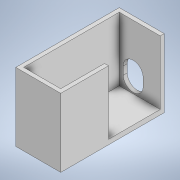
# Autodesk Inventor part: GoProCase
Saved by Autodesk Inventor 2020 (Build 240168000, 168)
## iProperties
Created: 2020-02-15
Part Number: GoProCase
Material: Generic
Document SubType Name: Modeling
Designer: maple
Density: 1 g/cm^3
Appearance: Default
Author: maple
Autodesk Inventor part; units mm, degrees
ref_plane "YZ Plane" through (0, 0, 0) normal (1, 0, 0) x (0, 1, 0)
ref_plane "XZ Plane" through (0, 0, 0) normal (0, 1, 0) x (-1, 0, 0)
ref_plane "XY Plane" through (0, 0, 0) normal (0, 0, 1) x (1, 0, 0)
sketch "Sketch1" plane through (0, 0, 0) normal (0, 1, 0) x (-1, 0, 0)
  line L0 (0, 0) -> (-28.702, 0)
  line L1 (-28.702, 0) -> (-28.702, -66.04)
  line L2 (-28.702, -66.04) -> (0, -66.04)
  line L3 (0, -66.04) -> (0, 0)
  dimension "d0" = 28.702
  dimension "d1" = 66.04
  constraints: 8 end point, 2 parallel, 1 horizontal, 1 perpendicular
  measures "d0" distance of L2.end L1.end
  measures "d1" distance of L1.end L0.end
extrude "Extrusion1" add sketch "Sketch1" along normal blind 3.048
sketch "Sketch2" plane through (0, 3.048, 0) normal (0, 1, 0) x (1, 0, 0)
  line L0 (0, 66.04) -> (0, 0) projected
  line L1 (28.702, 66.04) -> (0, 66.04) projected
  line L2 (0, 0) -> (2.54, 0)
  line L3 (2.54, 0) -> (2.54, 66.04)
  line L4 (2.54, 66.04) -> (0, 66.04)
  line L5 (0, 66.04) -> (0, 0)
  line L6 (28.702, 0) -> (28.702, 66.04) projected
  line L7 (28.702, 0) -> (2.54, 0)
  line L8 (2.54, 0) -> (2.54, 2.54)
  line L9 (2.54, 2.54) -> (28.702, 2.54)
  line L10 (28.702, 2.54) -> (28.702, 0)
  line L11 (2.54, 66.04) -> (28.702, 66.04)
  line L12 (28.702, 66.04) -> (28.702, 63.5)
  line L13 (28.702, 63.5) -> (2.54, 63.5)
  line L14 (2.54, 63.5) -> (2.54, 66.04)
  line L15 (28.702, 2.54) -> (26.162, 2.54)
  line L16 (26.162, 2.54) -> (26.162, 30.48)
  line L17 (26.162, 30.48) -> (28.702, 30.48)
  line L18 (28.702, 30.48) -> (28.702, 2.54)
  dimension "d4" = 2.54
  dimension "d5" = 2.54
  dimension "d6" = 2.54
  dimension "d7" = 2.54
  dimension "d8" = 27.94
  constraints: 32 end point, 8 parallel, 4 horizontal, 4 perpendicular, 3 point on line
  measures "d4" distance of L4.end L3.end
  measures "d5" distance of L7.end L8.end
  measures "d6" distance of L11.end L12.end
  measures "d7" distance of L16.end L17.end
  measures "d8" distance of L15.end L16.end
extrude "Extrusion2" add sketch "Sketch2" along normal blind 40.64 contours L1 L3 L2 L0 | L1 L6 L13 L3 | L3 L9 L6 L7 | L16 L17 L6 L9
sketch "Sketch3" plane through (28.702, 0, -66.04) normal (0, 0, -1) x (-1, 0, 0)
  line L0 (28.702, 0) -> (23.622, 0)
  line L1 (23.622, 0) -> (23.622, 3.81)
  line L2 (23.622, 3.81) -> (28.702, 3.81)
  line L3 (28.702, 3.81) -> (28.702, 0)
  line L4 (23.622, 3.81) -> (10.922, 3.81)
  line L5 (10.922, 3.81) -> (10.922, 21.59)
  line L6 (10.922, 21.59) -> (23.622, 21.59)
  line L7 (23.622, 21.59) -> (23.622, 3.81)
  dimension "d11" = 5.08
  dimension "d12" = 3.81
  dimension "d13" = 12.7
  dimension "d14" = 17.78
  constraints: 16 end point, 4 parallel, 2 horizontal, 2 perpendicular
  measures "d11" distance of L1.end L2.end
  measures "d12" distance of L0.end L1.end
  measures "d13" distance of L5.end L6.end
  measures "d14" distance of L4.end L5.end
extrude "Extrusion3" cut sketch "Sketch3" against normal blind 2.54 contours L4 L5 L6 L7
fillet "Fillet1" radius 6.35 4 edges at (17.78, 21.59, -64.77) (5.08, 21.59, -64.77) (5.08, 3.81, -64.77) (17.78, 3.81, -64.77)
body "Solid1"
